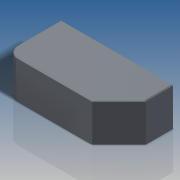
# Autodesk Inventor part: 11030-LtBluishGray
Saved by Autodesk Inventor 2016 SP2 (Build 200236200, 236)
## iProperties
Created: 2015-08-19
Part Number: 11030-LtBluishGray
Material: ABS Plastic
Document SubType Name: Modeling
Designer: D. Kohfeld
Mass: 0.586718 g
Surface Area: 4.31038 cm^2
Volume: 0.553507 cm^3
Density: 1.06 g/cm^3
Appearance: LtBluishGray
Author: D. Kohfeld
Autodesk Inventor part; units mm, degrees
ref_plane "YZ Plane" through (0, 0, 0) normal (1, 0, 0) x (0, 1, 0)
ref_plane "XZ Plane" through (0, 0, 0) normal (0, 1, 0) x (-1, 0, 0)
ref_plane "XY Plane" through (0, 0, 0) normal (0, 0, 1) x (1, 0, 0)
sketch "Sketch2" plane through (0, 0, 0) normal (0, 1, 0) x (-1, 0, 0)
  line L0 (-7.64, 0.08) -> (-7.64, -3.72)
  line L1 (-7.64, -3.72) -> (7.64, -3.72)
  line L2 (7.64, -3.72) -> (7.64, 2.12)
  arc A0 (7.64, 2.12) -> (6.04, 3.72) centre (6.04, 2.12) ccw
  line L3 (6.04, 3.72) -> (-4, 3.72)
  line L4 (-4, 3.72) -> (-7.64, 0.08)
  line L5 (0, -3.72) -> (0, 3.72) construction
  point P0 (0, 0)
  point P1 (0, 0)
  dimension "d0" = 7.44
  dimension "d1" = 15.28
  dimension "d2" = 1.6
  dimension "d3" = 3.64
  dimension "d4" = 3.64
  constraints: 12 end point, 3 vertical, 2 horizontal, 2 midpoint, 2 point on circle, 2 tangent, 1 centre point, 1 coincident, 1 point on line
  measures "d0" distance between parallel lines of L1 L3
  measures "d1" distance between parallel lines of L2 L0
  measures "d2" radius of A0
  measures "d3" distance from line of L3.end L0
  measures "d4" horizontal distance of L3.end L0.start
extrude "Extrusion1" add sketch "Sketch2" along normal mid plane 5.2
fillet "Fillet1" radius 0.12 4 edges at (4, 0, 3.72) (7.64, 0, 0.08) (7.64, 0, -3.72) (-7.64, 0, -3.72)
chamfer "Chamfer2" distance 0.12 angle 45 10 edges at (-7.1714, 2.6, 3.2514) (-1.0449, 2.6, 3.72) (3.9962, 2.6, 3.7109) (5.82, 2.6, 1.9) (7.6309, 2.6, 0.0762) (7.64, 2.6, -1.7849) (7.6049, 2.6, -3.6849) (0, 2.6, -3.72) (-7.6049, 2.6, -3.6849) (-7.64, 2.6, -0.74)
equation "\"d4\" = d3"
body "Solid1"
